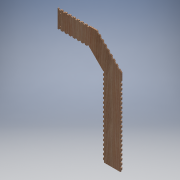
# Autodesk Inventor part: Leg
Saved by Autodesk Inventor 2019 (Build 230136000, 136)
## iProperties
Created: 2019-01-14
Part Number: Leg
Material: Wood (Birch)
Document SubType Name: Modeling
Designer: nxgam
Density: 0.55 g/cm^3
Appearance: Birch - Natural Polished
Author: nxgam
Autodesk Inventor part; units mm, degrees
(part 1 of 2)
ref_plane "YZ Plane" through (0, 0, 0) normal (1, 0, 0) x (0, 1, 0)
ref_plane "XZ Plane" through (0, 0, 0) normal (0, 1, 0) x (-1, 0, 0)
ref_plane "XY Plane" through (0, 0, 0) normal (0, 0, 1) x (1, 0, 0)
sketch "Sketch1" plane through (0, 0, 0) normal (0, 0, 1) x (1, 0, 0)
  line L0 (223.52, 0) -> (314.96, 0)
  line L1 (314.96, 0) -> (314.96, 396.2274)
  line L2 (314.96, 396.2274) -> (223.52, 396.2274)
  line L3 (223.52, 396.2274) -> (223.52, 0)
  line L4 (223.52, 396.2274) -> (154.9528, 464.7946)
  line L5 (154.9528, 464.7946) -> (219.6107, 529.4524)
  line L6 (219.6107, 529.4524) -> (314.96, 434.1031)
  line L7 (314.96, 434.1031) -> (314.96, 396.2274)
  line L8 (154.9528, 464.7946) -> (0, 464.7946)
  line L9 (0, 464.7946) -> (0, 556.2346)
  line L10 (0, 556.2346) -> (192.8285, 556.2346)
  line L11 (192.8285, 556.2346) -> (219.6107, 529.4524)
  circle A0 centre (0, 510.5146) radius 19.05
  line L12 (0, 0) -> (0, 464.7946) construction
  line L13 (0, 0) -> (223.52, 0) construction
  dimension "d0" = 91.44
  dimension "d2" = 91.44
  dimension "d3" = 135
  dimension "d4" = 91.44
  dimension "d5" = 38.1
  dimension "d6" = 556.2346
  dimension "d7" = 223.52
  dimension "d24" = 172.72
  constraints: 28 end point, 7 perpendicular, 4 collinear, 2 horizontal, 2 parallel, 2 point on line, 1 centre point, 1 midpoint
  measures "d0" distance of L2.end L1.end
  measures "d2" distance between parallel lines of L6 L4
  measures "d3" angle of L4 L3
  measures "d4" distance between parallel lines of L10 L8
  measures "d5" diameter of A0
  measures "d6" distance between parallel lines of L10 L13
  measures "d7" distance between parallel lines of L12 L3
  measures "d24" distance of L6.end L10.end
extrude "Extrusion1" add sketch "Sketch1" along normal blind 5.08 contours L3 L2 L1 L0 | L4 L5 L6 L7 L2 | L8 L9 A0 L10 L11 L5 | L9 A0 picked at (5.3722, 505.7092)
sketch "Sketch3" plane through (0, 0, 5.08) normal (0, 0, 1) x (1, 0, 0)
  line L0 (0, 464.7946) -> (154.9528, 464.7946) projected
  line L1 (0, 464.7946) -> (10.16, 464.7946)
  line L2 (10.16, 464.7946) -> (10.16, 469.8746)
  line L3 (10.16, 469.8746) -> (0, 469.8746)
  line L4 (0, 469.8746) -> (0, 464.7946)
  line L5 (192.8285, 556.2346) -> (0, 556.2346) construction
  line L6 (0, 556.2346) -> (0, 464.7946) construction
  line L7 (0, 510.5146) -> (154.9528, 510.5146) construction
  line L8 (154.9528, 510.5146) -> (154.9528, 464.7946) construction
  line L9 (192.8285, 556.2346) -> (154.9528, 464.7946) construction
  line L10 (154.9528, 464.7946) -> (223.52, 396.2274) construction
  line L11 (314.96, 0) -> (314.96, 434.1031) construction
  line L12 (223.52, 396.2274) -> (314.96, 434.1031) construction
  line L13 (314.96, 434.1031) -> (192.8285, 556.2346) construction
  line L14 (0, 556.2346) -> (0, 464.7946) construction
  line L15 (0, 464.7946) -> (154.9528, 464.7946) construction
  line L16 (154.9528, 464.7946) -> (223.52, 396.2274) construction
  line L17 (223.52, 396.2274) -> (223.52, 0) construction
  line L18 (223.52, 0) -> (314.96, 0) construction
  line L19 (314.96, 0) -> (314.96, 434.1031) construction
  line L20 (314.96, 434.1031) -> (192.8285, 556.2346) construction
  line L21 (192.8285, 556.2346) -> (0, 556.2346) construction
  line L22 (30.48, 464.7946) -> (30.48, 469.8746)
  line L23 (20.32, 464.7946) -> (30.48, 464.7946)
  line L24 (20.32, 469.8746) -> (20.32, 464.7946)
  line L25 (30.48, 469.8746) -> (20.32, 469.8746)
  line L26 (50.8, 464.7946) -> (50.8, 469.8746)
  line L27 (40.64, 464.7946) -> (50.8, 464.7946)
  line L28 (40.64, 469.8746) -> (40.64, 464.7946)
  line L29 (50.8, 469.8746) -> (40.64, 469.8746)
  line L30 (71.12, 464.7946) -> (71.12, 469.8746)
  line L31 (60.96, 464.7946) -> (71.12, 464.7946)
  line L32 (60.96, 469.8746) -> (60.96, 464.7946)
  line L33 (71.12, 469.8746) -> (60.96, 469.8746)
  line L34 (91.44, 464.7946) -> (91.44, 469.8746)
  line L35 (81.28, 464.7946) -> (91.44, 464.7946)
  line L36 (81.28, 469.8746) -> (81.28, 464.7946)
  line L37 (91.44, 469.8746) -> (81.28, 469.8746)
  line L38 (111.76, 464.7946) -> (111.76, 469.8746)
  line L39 (101.6, 464.7946) -> (111.76, 464.7946)
  line L40 (101.6, 469.8746) -> (101.6, 464.7946)
  line L41 (111.76, 469.8746) -> (101.6, 469.8746)
  line L42 (132.08, 464.7946) -> (132.08, 469.8746)
  line L43 (121.92, 464.7946) -> (132.08, 464.7946)
  line L44 (121.92, 469.8746) -> (121.92, 464.7946)
  line L45 (132.08, 469.8746) -> (121.92, 469.8746)
  line L46 (152.4, 464.7946) -> (152.4, 469.8746)
  line L47 (142.24, 464.7946) -> (152.4, 464.7946)
  line L48 (142.24, 469.8746) -> (142.24, 464.7946)
  line L49 (152.4, 469.8746) -> (142.24, 469.8746)
  line L50 (172.72, 464.7946) -> (172.72, 469.8746)
  line L51 (162.56, 464.7946) -> (172.72, 464.7946)
  line L52 (162.56, 469.8746) -> (162.56, 464.7946)
  line L53 (172.72, 469.8746) -> (162.56, 469.8746)
  line L54 (193.04, 464.7946) -> (193.04, 469.8746)
  line L55 (182.88, 464.7946) -> (193.04, 464.7946)
  line L56 (182.88, 469.8746) -> (182.88, 464.7946)
  line L57 (193.04, 469.8746) -> (182.88, 469.8746)
  line L58 (213.36, 464.7946) -> (213.36, 469.8746)
  line L59 (203.2, 464.7946) -> (213.36, 464.7946)
  line L60 (203.2, 469.8746) -> (203.2, 464.7946)
  line L61 (213.36, 469.8746) -> (203.2, 469.8746)
  line L62 (233.68, 464.7946) -> (233.68, 469.8746)
  line L63 (223.52, 464.7946) -> (233.68, 464.7946)
  line L64 (223.52, 469.8746) -> (223.52, 464.7946)
  line L65 (233.68, 469.8746) -> (223.52, 469.8746)
  line L66 (0, 556.2346) -> (10.16, 556.2346)
  line L67 (10.16, 556.2346) -> (10.16, 551.1546)
  line L68 (10.16, 551.1546) -> (0, 551.1546)
  line L69 (0, 551.1546) -> (0, 556.2346)
  line L70 (30.48, 556.2346) -> (30.48, 551.1546)
  line L71 (20.32, 556.2346) -> (30.48, 556.2346)
  line L72 (20.32, 551.1546) -> (20.32, 556.2346)
  line L73 (30.48, 551.1546) -> (20.32, 551.1546)
  line L74 (50.8, 556.2346) -> (50.8, 551.1546)
  line L75 (40.64, 556.2346) -> (50.8, 556.2346)
  line L76 (40.64, 551.1546) -> (40.64, 556.2346)
  line L77 (50.8, 551.1546) -> (40.64, 551.1546)
  line L78 (71.12, 556.2346) -> (71.12, 551.1546)
  line L79 (60.96, 556.2346) -> (71.12, 556.2346)
  line L80 (60.96, 551.1546) -> (60.96, 556.2346)
  line L81 (71.12, 551.1546) -> (60.96, 551.1546)
  line L82 (91.44, 556.2346) -> (91.44, 551.1546)
  line L83 (81.28, 556.2346) -> (91.44, 556.2346)
  line L84 (81.28, 551.1546) -> (81.28, 556.2346)
  line L85 (91.44, 551.1546) -> (81.28, 551.1546)
  line L86 (111.76, 556.2346) -> (111.76, 551.1546)
  line L87 (101.6, 556.2346) -> (111.76, 556.2346)
  line L88 (101.6, 551.1546) -> (101.6, 556.2346)
  line L89 (111.76, 551.1546) -> (101.6, 551.1546)
  line L90 (132.08, 556.2346) -> (132.08, 551.1546)
  line L91 (121.92, 556.2346) -> (132.08, 556.2346)
  line L92 (121.92, 551.1546) -> (121.92, 556.2346)
  line L93 (132.08, 551.1546) -> (121.92, 551.1546)
  line L94 (152.4, 556.2346) -> (152.4, 551.1546)
  line L95 (142.24, 556.2346) -> (152.4, 556.2346)
  line L96 (142.24, 551.1546) -> (142.24, 556.2346)
  line L97 (152.4, 551.1546) -> (142.24, 551.1546)
  line L98 (172.72, 556.2346) -> (172.72, 551.1546)
  line L99 (162.56, 556.2346) -> (172.72, 556.2346)
  line L100 (162.56, 551.1546) -> (162.56, 556.2346)
  line L101 (172.72, 551.1546) -> (162.56, 551.1546)
  line L102 (193.04, 556.2346) -> (193.04, 551.1546)
  line L103 (182.88, 556.2346) -> (193.04, 556.2346)
  line L104 (182.88, 551.1546) -> (182.88, 556.2346)
  line L105 (193.04, 551.1546) -> (182.88, 551.1546)
  line L106 (213.36, 556.2346) -> (213.36, 551.1546)
  line L107 (203.2, 556.2346) -> (213.36, 556.2346)
  line L108 (203.2, 551.1546) -> (203.2, 556.2346)
  line L109 (213.36, 551.1546) -> (203.2, 551.1546)
  line L110 (233.68, 556.2346) -> (233.68, 551.1546)
  line L111 (223.52, 556.2346) -> (233.68, 556.2346)
  line L112 (223.52, 551.1546) -> (223.52, 556.2346)
  line L113 (233.68, 551.1546) -> (223.52, 551.1546)
  line L114 (223.52, 0) -> (314.96, 0) construction
  line L115 (269.24, 0) -> (269.24, 396.2274) construction
  line L116 (269.24, 396.2274) -> (223.52, 396.2274) construction
  line L117 (223.52, 396.2274) -> (228.6, 396.2274)
  line L118 (228.6, 396.2274) -> (228.6, 386.0674)
  line L119 (228.6, 386.0674) -> (223.52, 386.0674)
  line L120 (223.52, 386.0674) -> (223.52, 396.2274)
  line L121 (223.52, 375.9074) -> (228.6, 375.9074)
  line L122 (228.6, 375.9074) -> (228.6, 365.7474)
  line L123 (228.6, 365.7474) -> (223.52, 365.7474)
  line L124 (223.52, 365.7474) -> (223.52, 375.9074)
  line L125 (223.52, 355.5874) -> (228.6, 355.5874)
  line L126 (228.6, 355.5874) -> (228.6, 345.4274)
  line L127 (228.6, 345.4274) -> (223.52, 345.4274)
  line L128 (223.52, 345.4274) -> (223.52, 355.5874)
  line L129 (223.52, 335.2674) -> (228.6, 335.2674)
  line L130 (228.6, 335.2674) -> (228.6, 325.1074)
  line L131 (228.6, 325.1074) -> (223.52, 325.1074)
  line L132 (223.52, 325.1074) -> (223.52, 335.2674)
  line L133 (223.52, 314.9474) -> (228.6, 314.9474)
  line L134 (228.6, 314.9474) -> (228.6, 304.7874)
  line L135 (228.6, 304.7874) -> (223.52, 304.7874)
  line L136 (223.52, 304.7874) -> (223.52, 314.9474)
  line L137 (223.52, 294.6274) -> (228.6, 294.6274)
  line L138 (228.6, 294.6274) -> (228.6, 284.4674)
  line L139 (228.6, 284.4674) -> (223.52, 284.4674)
  line L140 (223.52, 284.4674) -> (223.52, 294.6274)
  line L141 (223.52, 274.3074) -> (228.6, 274.3074)
  line L142 (228.6, 274.3074) -> (228.6, 264.1474)
  line L143 (228.6, 264.1474) -> (223.52, 264.1474)
  line L144 (223.52, 264.1474) -> (223.52, 274.3074)
  line L145 (223.52, 253.9874) -> (228.6, 253.9874)
  line L146 (228.6, 253.9874) -> (228.6, 243.8274)
  line L147 (228.6, 243.8274) -> (223.52, 243.8274)
  line L148 (223.52, 243.8274) -> (223.52, 253.9874)
  line L149 (223.52, 233.6674) -> (228.6, 233.6674)
  line L150 (228.6, 233.6674) -> (228.6, 223.5074)
  line L151 (228.6, 223.5074) -> (223.52, 223.5074)
  line L152 (223.52, 223.5074) -> (223.52, 233.6674)
  line L153 (223.52, 213.3474) -> (228.6, 213.3474)
  line L154 (228.6, 213.3474) -> (228.6, 203.1874)
  line L155 (228.6, 203.1874) -> (223.52, 203.1874)
  line L156 (223.52, 203.1874) -> (223.52, 213.3474)
  line L157 (223.52, 193.0274) -> (228.6, 193.0274)
  line L158 (228.6, 193.0274) -> (228.6, 182.8674)
  line L159 (228.6, 182.8674) -> (223.52, 182.8674)
  line L160 (223.52, 182.8674) -> (223.52, 193.0274)
  line L161 (223.52, 172.7074) -> (228.6, 172.7074)
  line L162 (228.6, 172.7074) -> (228.6, 162.5474)
  line L163 (228.6, 162.5474) -> (223.52, 162.5474)
  line L164 (223.52, 162.5474) -> (223.52, 172.7074)
  line L165 (223.52, 152.3874) -> (228.6, 152.3874)
  line L166 (228.6, 152.3874) -> (228.6, 142.2274)
  line L167 (228.6, 142.2274) -> (223.52, 142.2274)
  line L168 (223.52, 142.2274) -> (223.52, 152.3874)
  line L169 (223.52, 132.0674) -> (228.6, 132.0674)
  line L170 (228.6, 132.0674) -> (228.6, 121.9074)
  line L171 (228.6, 121.9074) -> (223.52, 121.9074)
  line L172 (223.52, 121.9074) -> (223.52, 132.0674)
  line L173 (223.52, 111.7474) -> (228.6, 111.7474)
  line L174 (228.6, 111.7474) -> (228.6, 101.5874)
  line L175 (228.6, 101.5874) -> (223.52, 101.5874)
  line L176 (223.52, 101.5874) -> (223.52, 111.7474)
  line L177 (223.52, 91.4274) -> (228.6, 91.4274)
  line L178 (228.6, 91.4274) -> (228.6, 81.2674)
  line L179 (228.6, 81.2674) -> (223.52, 81.2674)
  line L180 (223.52, 81.2674) -> (223.52, 91.4274)
  line L181 (314.96, 396.2274) -> (309.88, 396.2274)
  line L182 (309.88, 396.2274) -> (309.88, 386.0674)
  line L183 (309.88, 386.0674) -> (314.96, 386.0674)
  line L184 (314.96, 386.0674) -> (314.96, 396.2274)
  line L185 (314.96, 375.9074) -> (309.88, 375.9074)
  line L186 (309.88, 375.9074) -> (309.88, 365.7474)
  line L187 (309.88, 365.7474) -> (314.96, 365.7474)
  line L188 (314.96, 365.7474) -> (314.96, 375.9074)
  line L189 (314.96, 355.5874) -> (309.88, 355.5874)
  line L190 (309.88, 355.5874) -> (309.88, 345.4274)
  line L191 (309.88, 345.4274) -> (314.96, 345.4274)
  line L192 (314.96, 345.4274) -> (314.96, 355.5874)
  line L193 (314.96, 335.2674) -> (309.88, 335.2674)
  line L194 (309.88, 335.2674) -> (309.88, 325.1074)
  line L195 (309.88, 325.1074) -> (314.96, 325.1074)
  line L196 (314.96, 325.1074) -> (314.96, 335.2674)
  line L197 (314.96, 314.9474) -> (309.88, 314.9474)
  line L198 (309.88, 314.9474) -> (309.88, 304.7874)
  line L199 (309.88, 304.7874) -> (314.96, 304.7874)
  line L200 (314.96, 304.7874) -> (314.96, 314.9474)
  line L201 (314.96, 294.6274) -> (309.88, 294.6274)
  line L202 (309.88, 294.6274) -> (309.88, 284.4674)
  line L203 (309.88, 284.4674) -> (314.96, 284.4674)
  line L204 (314.96, 284.4674) -> (314.96, 294.6274)
  line L205 (314.96, 274.3074) -> (309.88, 274.3074)
  line L206 (309.88, 274.3074) -> (309.88, 264.1474)
  line L207 (309.88, 264.1474) -> (314.96, 264.1474)
  line L208 (314.96, 264.1474) -> (314.96, 274.3074)
  line L209 (314.96, 253.9874) -> (309.88, 253.9874)
  line L210 (309.88, 253.9874) -> (309.88, 243.8274)
  line L211 (309.88, 243.8274) -> (314.96, 243.8274)
  line L212 (314.96, 243.8274) -> (314.96, 253.9874)
  line L213 (314.96, 233.6674) -> (309.88, 233.6674)
  line L214 (309.88, 233.6674) -> (309.88, 223.5074)
  line L215 (309.88, 223.5074) -> (314.96, 223.5074)
  line L216 (314.96, 223.5074) -> (314.96, 233.6674)
  line L217 (314.96, 213.3474) -> (309.88, 213.3474)
  line L218 (309.88, 213.3474) -> (309.88, 203.1874)
  line L219 (309.88, 203.1874) -> (314.96, 203.1874)
  line L220 (314.96, 203.1874) -> (314.96, 213.3474)
  line L221 (314.96, 193.0274) -> (309.88, 193.0274)
  line L222 (309.88, 193.0274) -> (309.88, 182.8674)
  line L223 (309.88, 182.8674) -> (314.96, 182.8674)
  line L224 (314.96, 182.8674) -> (314.96, 193.0274)
  line L225 (314.96, 172.7074) -> (309.88, 172.7074)
  line L226 (309.88, 172.7074) -> (309.88, 162.5474)
  line L227 (309.88, 162.5474) -> (314.96, 162.5474)
  line L228 (314.96, 162.5474) -> (314.96, 172.7074)
  line L229 (314.96, 152.3874) -> (309.88, 152.3874)
  line L230 (309.88, 152.3874) -> (309.88, 142.2274)
  line L231 (309.88, 142.2274) -> (314.96, 142.2274)
  line L232 (314.96, 142.2274) -> (314.96, 152.3874)
  line L233 (314.96, 132.0674) -> (309.88, 132.0674)
  line L234 (309.88, 132.0674) -> (309.88, 121.9074)
  line L235 (309.88, 121.9074) -> (314.96, 121.9074)
  line L236 (314.96, 121.9074) -> (314.96, 132.0674)
  line L237 (314.96, 111.7474) -> (309.88, 111.7474)
  line L238 (309.88, 111.7474) -> (309.88, 101.5874)
  line L239 (309.88, 101.5874) -> (314.96, 101.5874)
  line L240 (314.96, 101.5874) -> (314.96, 111.7474)
  line L241 (314.96, 91.4274) -> (309.88, 91.4274)
  line L242 (309.88, 91.4274) -> (309.88, 81.2674)
  line L243 (309.88, 81.2674) -> (314.96, 81.2674)
  line L244 (314.96, 81.2674) -> (314.96, 91.4274)
  line L245 (196.4206, 552.6425) -> (203.6048, 545.4583)
  line L246 (203.6048, 545.4583) -> (200.0127, 541.8662)
  line L247 (200.0127, 541.8662) -> (192.8285, 549.0504)
  line L248 (192.8285, 549.0504) -> (196.4206, 552.6425)
  line L249 (207.1969, 534.682) -> (210.789, 538.2741)
  line L250 (214.3811, 527.4978) -> (207.1969, 534.682)
  line L251 (210.789, 538.2741) -> (217.9732, 531.0899)
  line L252 (217.9732, 531.0899) -> (214.3811, 527.4978)
  line L253 (221.5653, 520.3136) -> (225.1574, 523.9057)
  line L254 (228.7495, 513.1294) -> (221.5653, 520.3136)
  line L255 (225.1574, 523.9057) -> (232.3416, 516.7215)
  line L256 (232.3416, 516.7215) -> (228.7495, 513.1294)
  line L257 (235.9337, 505.9452) -> (239.5258, 509.5373)
  line L258 (243.118, 498.761) -> (235.9337, 505.9452)
  line L259 (239.5258, 509.5373) -> (246.7101, 502.3531)
  line L260 (246.7101, 502.3531) -> (243.118, 498.761)
  line L261 (250.3022, 491.5768) -> (253.8943, 495.1689)
  line L262 (257.4864, 484.3926) -> (250.3022, 491.5768)
  line L263 (253.8943, 495.1689) -> (261.0785, 487.9847)
  line L264 (261.0785, 487.9847) -> (257.4864, 484.3926)
  line L265 (264.6706, 477.2083) -> (268.2627, 480.8004)
  line L266 (271.8548, 470.0241) -> (264.6706, 477.2083)
  line L267 (268.2627, 480.8004) -> (275.4469, 473.6162)
  line L268 (275.4469, 473.6162) -> (271.8548, 470.0241)
  line L269 (279.039, 462.8399) -> (282.6311, 466.432)
  line L270 (286.2232, 455.6557) -> (279.039, 462.8399)
  line L271 (282.6311, 466.432) -> (289.8153, 459.2478)
  line L272 (289.8153, 459.2478) -> (286.2232, 455.6557)
  line L273 (293.4074, 448.4715) -> (296.9995, 452.0636)
  line L274 (300.5916, 441.2873) -> (293.4074, 448.4715)
  line L275 (296.9995, 452.0636) -> (304.1837, 444.8794)
  line L276 (304.1837, 444.8794) -> (300.5916, 441.2873)
  point P0 (0, 0)
  point P1 (0, 556.2346)
  point P2 (207.1969, 541.8662)
  point P3 (207.1969, 541.8662)
  point P4 (207.1969, 541.8662)
  point P5 (207.1969, 541.8662)
  point P6 (221.5653, 527.4978)
  point P7 (221.5653, 527.4978)
  point P8 (221.5653, 527.4978)
  point P9 (221.5653, 527.4978)
  point P10 (235.9337, 513.1294)
  point P11 (235.9337, 513.1294)
  point P12 (235.9337, 513.1294)
  point P13 (235.9337, 513.1294)
  point P14 (250.3022, 498.761)
  point P15 (250.3022, 498.761)
  point P16 (250.3022, 498.761)
  point P17 (250.3022, 498.761)
  point P18 (264.6706, 484.3926)
  point P19 (264.6706, 484.3926)
  point P20 (264.6706, 484.3926)
  point P21 (264.6706, 484.3926)
  point P22 (279.039, 470.0241)
  point P23 (279.039, 470.0241)
  point P24 (279.039, 470.0241)
  point P25 (279.039, 470.0241)
  point P26 (293.4074, 455.6557)
  point P27 (293.4074, 455.6557)
  point P28 (293.4074, 455.6557)
  point P29 (293.4074, 455.6557)
  dimension "d14" = 10.16
  dimension "d15" = 5.08
  dimension "d18" = 20.32
  dimension "d34" = 5.08
  dimension "d35" = 10.16
  dimension "d38" = 20.32
  dimension "d47" = 5.08
  dimension "d48" = 10.16
  dimension "d49" = 5.08
  dimension "d52" = 20.32
  constraints: 528 end point, 125 symmetric about line, 6 parallel, 6 perpendicular, 4 horizontal, 2 midpoint, 2 point on line, 2 vertical, 304 other
  measures "d14" distance of L3.end L2.end
  measures "d15" distance of L2.end L1.end
  measures "d18" distance of L0.start L23.start
  measures "d34" distance of L118.end L119.end
  measures "d35" distance of L117.end L118.end
  measures "d38" distance of L16.end L121.start
  measures "d47" distance of L245.end L246.end
  measures "d48" distance of L246.end L247.end
  measures "d49" distance from line of L20.end L248
  measures "d52" distance of L13.end point (207.197, 541.866)
extrude "Extrusion3" cut sketch "Sketch3" against normal blind 5.08
thicken "Thicken1" operation add thickness 5.08 both sides no extend neighbours yes toward (-1, 0, 0) faces at (0, 524.0613, 1.6933)
sketch "Sketch5" plane through (0, 0, 5.08) normal (0, 0, 1) x (1, 0, 0)
  line L0 (279.039, 462.8399) -> (282.6311, 466.432) projected
  line L1 (282.6311, 466.432) -> (275.4469, 473.6162) projected
  line L2 (275.4469, 473.6162) -> (271.8548, 470.0241) projected
  line L3 (271.8548, 470.0241) -> (264.6706, 477.2083) projected
  line L4 (264.6706, 477.2083) -> (268.2627, 480.8004) projected
  line L5 (268.2627, 480.8004) -> (261.0785, 487.9847) projected
  line L6 (261.0785, 487.9847) -> (257.4864, 484.3926) projected
  line L7 (257.4864, 484.3926) -> (250.3022, 491.5768) projected
  line L8 (250.3022, 491.5768) -> (253.8943, 495.1689) projected
  line L9 (253.8943, 495.1689) -> (246.7101, 502.3531) projected
  line L10 (246.7101, 502.3531) -> (243.118, 498.761) projected
  line L11 (243.118, 498.761) -> (235.9337, 505.9452) projected
  line L12 (235.9337, 505.9452) -> (239.5258, 509.5373) projected
  line L13 (239.5258, 509.5373) -> (232.3416, 516.7215) projected
  line L14 (232.3416, 516.7215) -> (228.7495, 513.1294) projected
  line L15 (228.7495, 513.1294) -> (221.5653, 520.3136) projected
  line L16 (221.5653, 520.3136) -> (225.1574, 523.9057) projected
  line L17 (225.1574, 523.9057) -> (217.9732, 531.0899) projected
  line L18 (217.9732, 531.0899) -> (214.3811, 527.4978) projected
  line L19 (214.3811, 527.4978) -> (207.1969, 534.682) projected
  line L20 (207.1969, 534.682) -> (210.789, 538.2741) projected
  line L21 (210.789, 538.2741) -> (203.6048, 545.4583) projected
  line L22 (203.6048, 545.4583) -> (200.0127, 541.8662) projected
  line L23 (200.0127, 541.8662) -> (192.8285, 549.0504) projected
  line L24 (192.8285, 549.0504) -> (196.4206, 552.6425) projected
  line L25 (196.4206, 552.6425) -> (193.04, 556.0231) projected
  line L26 (193.04, 556.0231) -> (193.04, 551.1546) projected
  line L27 (193.04, 551.1546) -> (182.88, 551.1546) projected
  line L28 (182.88, 551.1546) -> (182.88, 556.2346) projected
  line L29 (182.88, 556.2346) -> (172.72, 556.2346) projected
  line L30 (172.72, 556.2346) -> (172.72, 551.1546) projected
  line L31 (172.72, 551.1546) -> (162.56, 551.1546) projected
  line L32 (162.56, 551.1546) -> (162.56, 556.2346) projected
  line L33 (162.56, 556.2346) -> (152.4, 556.2346) projected
  line L34 (152.4, 556.2346) -> (152.4, 551.1546) projected
  line L35 (152.4, 551.1546) -> (142.24, 551.1546) projected
  line L36 (142.24, 551.1546) -> (142.24, 556.2346) projected
  line L37 (142.24, 556.2346) -> (132.08, 556.2346) projected
  line L38 (132.08, 556.2346) -> (132.08, 551.1546) projected
  line L39 (132.08, 551.1546) -> (121.92, 551.1546) projected
  line L40 (121.92, 551.1546) -> (121.92, 556.2346) projected
  line L41 (121.92, 556.2346) -> (111.76, 556.2346) projected
  line L42 (111.76, 556.2346) -> (111.76, 551.1546) projected
  line L43 (111.76, 551.1546) -> (101.6, 551.1546) projected
  line L44 (101.6, 551.1546) -> (101.6, 556.2346) projected
  line L45 (101.6, 556.2346) -> (91.44, 556.2346) projected
  line L46 (91.44, 556.2346) -> (91.44, 551.1546) projected
  line L47 (91.44, 551.1546) -> (81.28, 551.1546) projected
  line L48 (81.28, 551.1546) -> (81.28, 556.2346) projected
  line L49 (81.28, 556.2346) -> (71.12, 556.2346) projected
  line L50 (71.12, 556.2346) -> (71.12, 551.1546) projected
  line L51 (71.12, 551.1546) -> (60.96, 551.1546) projected
  line L52 (60.96, 551.1546) -> (60.96, 556.2346) projected
  line L53 (60.96, 556.2346) -> (50.8, 556.2346) projected
  line L54 (50.8, 556.2346) -> (50.8, 551.1546) projected
  line L55 (50.8, 551.1546) -> (40.64, 551.1546) projected
  line L56 (40.64, 551.1546) -> (40.64, 556.2346) projected
  line L57 (40.64, 556.2346) -> (30.48, 556.2346) projected
  line L58 (30.48, 556.2346) -> (30.48, 551.1546) projected
  line L59 (30.48, 551.1546) -> (20.32, 551.1546) projected
  line L60 (20.32, 551.1546) -> (20.32, 556.2346) projected
  line L61 (20.32, 556.2346) -> (10.16, 556.2346) projected
  line L62 (10.16, 556.2346) -> (10.16, 551.1546) projected
  line L63 (10.16, 551.1546) -> (-5.08, 551.1546) projected
  line L64 (-5.08, 551.1546) -> (-5.08, 469.8746) projected
  line L65 (-5.08, 469.8746) -> (10.16, 469.8746) projected
  line L66 (10.16, 469.8746) -> (10.16, 464.7946) projected
  line L67 (10.16, 464.7946) -> (20.32, 464.7946) projected
  line L68 (20.32, 464.7946) -> (20.32, 469.8746) projected
  line L69 (20.32, 469.8746) -> (30.48, 469.8746) projected
  line L70 (30.48, 469.8746) -> (30.48, 464.7946) projected
  line L71 (30.48, 464.7946) -> (40.64, 464.7946) projected
  line L72 (40.64, 464.7946) -> (40.64, 469.8746) projected
  line L73 (40.64, 469.8746) -> (50.8, 469.8746) projected
  line L74 (50.8, 469.8746) -> (50.8, 464.7946) projected
  line L75 (50.8, 464.7946) -> (60.96, 464.7946) projected
  line L76 (60.96, 464.7946) -> (60.96, 469.8746) projected
  line L77 (60.96, 469.8746) -> (71.12, 469.8746) projected
  line L78 (71.12, 469.8746) -> (71.12, 464.7946) projected
  line L79 (71.12, 464.7946) -> (81.28, 464.7946) projected
  line L80 (81.28, 464.7946) -> (81.28, 469.8746) projected
  line L81 (81.28, 469.8746) -> (91.44, 469.8746) projected
  line L82 (91.44, 469.8746) -> (91.44, 464.7946) projected
  line L83 (91.44, 464.7946) -> (101.6, 464.7946) projected
  line L84 (101.6, 464.7946) -> (101.6, 469.8746) projected
  line L85 (101.6, 469.8746) -> (111.76, 469.8746) projected
  line L86 (111.76, 469.8746) -> (111.76, 464.7946) projected
  line L87 (111.76, 464.7946) -> (121.92, 464.7946) projected
  line L88 (121.92, 464.7946) -> (121.92, 469.8746) projected
  line L89 (121.92, 469.8746) -> (132.08, 469.8746) projected
  line L90 (132.08, 469.8746) -> (132.08, 464.7946) projected
  line L91 (132.08, 464.7946) -> (142.24, 464.7946) projected
  line L92 (142.24, 464.7946) -> (142.24, 469.8746) projected
  line L93 (142.24, 469.8746) -> (152.4, 469.8746) projected
  line L94 (152.4, 469.8746) -> (152.4, 464.7946) projected
  line L95 (152.4, 464.7946) -> (154.9528, 464.7946) projected
  line L96 (162.56, 464.7946) -> (162.56, 469.8746) projected
  line L97 (162.56, 469.8746) -> (172.72, 469.8746) projected
  line L98 (172.72, 469.8746) -> (172.72, 464.7946) projected
  line L99 (182.88, 464.7946) -> (182.88, 469.8746) projected
  line L100 (182.88, 469.8746) -> (193.04, 469.8746) projected
  line L101 (193.04, 469.8746) -> (193.04, 464.7946) projected
  line L102 (203.2, 464.7946) -> (203.2, 469.8746) projected
  line L103 (203.2, 469.8746) -> (213.36, 469.8746) projected
  line L104 (213.36, 469.8746) -> (213.36, 464.7946) projected
  line L105 (223.52, 464.7946) -> (223.52, 469.8746) projected
  line L106 (223.52, 469.8746) -> (233.68, 469.8746) projected
  line L107 (233.68, 469.8746) -> (233.68, 464.7946) projected
  line L108 (154.9528, 464.7946) -> (223.52, 396.2274) projected
  line L109 (223.52, 396.2274) -> (228.6, 396.2274) projected
  line L110 (228.6, 396.2274) -> (228.6, 386.0674) projected
  line L111 (228.6, 386.0674) -> (223.52, 386.0674) projected
  line L112 (223.52, 386.0674) -> (223.52, 375.9074) projected
  line L113 (223.52, 375.9074) -> (228.6, 375.9074) projected
  line L114 (228.6, 375.9074) -> (228.6, 365.7474) projected
  line L115 (228.6, 365.7474) -> (223.52, 365.7474) projected
  line L116 (223.52, 365.7474) -> (223.52, 355.5874) projected
  line L117 (223.52, 355.5874) -> (228.6, 355.5874) projected
  line L118 (228.6, 355.5874) -> (228.6, 345.4274) projected
  line L119 (228.6, 345.4274) -> (223.52, 345.4274) projected
  line L120 (223.52, 345.4274) -> (223.52, 335.2674) projected
  line L121 (223.52, 335.2674) -> (228.6, 335.2674) projected
  line L122 (228.6, 335.2674) -> (228.6, 325.1074) projected
  line L123 (228.6, 325.1074) -> (223.52, 325.1074) projected
  line L124 (223.52, 325.1074) -> (223.52, 314.9474) projected
  line L125 (223.52, 314.9474) -> (228.6, 314.9474) projected
  line L126 (228.6, 314.9474) -> (228.6, 304.7874) projected
  line L127 (228.6, 304.7874) -> (223.52, 304.7874) projected
  line L128 (223.52, 304.7874) -> (223.52, 294.6274) projected
  line L129 (223.52, 294.6274) -> (228.6, 294.6274) projected
  line L130 (228.6, 294.6274) -> (228.6, 284.4674) projected
  line L131 (228.6, 284.4674) -> (223.52, 284.4674) projected
  line L132 (223.52, 284.4674) -> (223.52, 274.3074) projected
  line L133 (223.52, 274.3074) -> (228.6, 274.3074) projected
  line L134 (228.6, 274.3074) -> (228.6, 264.1474) projected
  line L135 (228.6, 264.1474) -> (223.52, 264.1474) projected
  line L136 (223.52, 264.1474) -> (223.52, 253.9874) projected
  line L137 (223.52, 253.9874) -> (228.6, 253.9874) projected
  line L138 (228.6, 253.9874) -> (228.6, 243.8274) projected
  line L139 (228.6, 243.8274) -> (223.52, 243.8274) projected
  line L140 (223.52, 243.8274) -> (223.52, 233.6674) projected
  line L141 (223.52, 233.6674) -> (228.6, 233.6674) projected
  line L142 (228.6, 233.6674) -> (228.6, 223.5074) projected
  line L143 (228.6, 223.5074) -> (223.52, 223.5074) projected
  line L144 (223.52, 223.5074) -> (223.52, 213.3474) projected
  line L145 (223.52, 213.3474) -> (228.6, 213.3474) projected
  line L146 (228.6, 213.3474) -> (228.6, 203.1874) projected
  line L147 (228.6, 203.1874) -> (223.52, 203.1874) projected
  line L148 (223.52, 203.1874) -> (223.52, 193.0274) projected
  line L149 (223.52, 193.0274) -> (228.6, 193.0274) projected
  line L150 (228.6, 193.0274) -> (228.6, 182.8674) projected
  line L151 (228.6, 182.8674) -> (223.52, 182.8674) projected
  line L152 (223.52, 182.8674) -> (223.52, 172.7074) projected
  line L153 (223.52, 172.7074) -> (228.6, 172.7074) projected
  line L154 (228.6, 172.7074) -> (228.6, 162.5474) projected
  line L155 (228.6, 162.5474) -> (223.52, 162.5474) projected
  line L156 (223.52, 162.5474) -> (223.52, 152.3874) projected
  line L157 (223.52, 152.3874) -> (228.6, 152.3874) projected
  line L158 (228.6, 152.3874) -> (228.6, 142.2274) projected
  line L159 (228.6, 142.2274) -> (223.52, 142.2274) projected
  line L160 (223.52, 142.2274) -> (223.52, 132.0674) projected
  line L161 (223.52, 132.0674) -> (228.6, 132.0674) projected
  line L162 (228.6, 132.0674) -> (228.6, 121.9074) projected
  line L163 (228.6, 121.9074) -> (223.52, 121.9074) projected
  line L164 (223.52, 121.9074) -> (223.52, 111.7474) projected
  line L165 (223.52, 111.7474) -> (228.6, 111.7474) projected
  line L166 (228.6, 111.7474) -> (228.6, 101.5874) projected
  line L167 (228.6, 101.5874) -> (223.52, 101.5874) projected
  line L168 (223.52, 101.5874) -> (223.52, 91.4274) projected
  line L169 (223.52, 91.4274) -> (228.6, 91.4274) projected
  line L170 (228.6, 91.4274) -> (228.6, 81.2674) projected
  line L171 (228.6, 81.2674) -> (223.52, 81.2674) projected
  line L172 (223.52, 81.2674) -> (223.52, 0) projected
  line L173 (223.52, 0) -> (314.96, 0) projected
  line L174 (314.96, 0) -> (314.96, 81.2674) projected
  line L175 (314.96, 81.2674) -> (309.88, 81.2674) projected
  line L176 (309.88, 81.2674) -> (309.88, 91.4274) projected
  line L177 (309.88, 91.4274) -> (314.96, 91.4274) projected
  line L178 (314.96, 91.4274) -> (314.96, 101.5874) projected
  line L179 (314.96, 101.5874) -> (309.88, 101.5874) projected
  line L180 (309.88, 101.5874) -> (309.88, 111.7474) projected
  line L181 (309.88, 111.7474) -> (314.96, 111.7474) projected
  line L182 (314.96, 111.7474) -> (314.96, 121.9074) projected
  line L183 (314.96, 121.9074) -> (309.88, 121.9074) projected
  line L184 (309.88, 121.9074) -> (309.88, 132.0674) projected
  line L185 (309.88, 132.0674) -> (314.96, 132.0674) projected
  line L186 (314.96, 132.0674) -> (314.96, 142.2274) projected
  line L187 (314.96, 142.2274) -> (309.88, 142.2274) projected
  line L188 (309.88, 142.2274) -> (309.88, 152.3874) projected
  line L189 (309.88, 152.3874) -> (314.96, 152.3874) projected
  line L190 (314.96, 152.3874) -> (314.96, 162.5474) projected
  line L191 (314.96, 162.5474) -> (309.88, 162.5474) projected
  line L192 (309.88, 162.5474) -> (309.88, 172.7074) projected
  line L193 (309.88, 172.7074) -> (314.96, 172.7074) projected
  line L194 (314.96, 172.7074) -> (314.96, 182.8674) projected
  line L195 (314.96, 182.8674) -> (309.88, 182.8674) projected
  line L196 (309.88, 182.8674) -> (309.88, 193.0274) projected
  line L197 (309.88, 193.0274) -> (314.96, 193.0274) projected
  line L198 (314.96, 193.0274) -> (314.96, 203.1874) projected
  line L199 (314.96, 203.1874) -> (309.88, 203.1874) projected
  line L200 (309.88, 203.1874) -> (309.88, 213.3474) projected
  line L201 (309.88, 213.3474) -> (314.96, 213.3474) projected
  line L202 (314.96, 213.3474) -> (314.96, 223.5074) projected
  line L203 (314.96, 223.5074) -> (309.88, 223.5074) projected
  line L204 (309.88, 223.5074) -> (309.88, 233.6674) projected
  line L205 (309.88, 233.6674) -> (314.96, 233.6674) projected
  line L206 (314.96, 233.6674) -> (314.96, 243.8274) projected
  line L207 (314.96, 243.8274) -> (309.88, 243.8274) projected
  line L208 (309.88, 243.8274) -> (309.88, 253.9874) projected
  line L209 (309.88, 253.9874) -> (314.96, 253.9874) projected
  line L210 (314.96, 253.9874) -> (314.96, 264.1474) projected
  line L211 (314.96, 264.1474) -> (309.88, 264.1474) projected
  line L212 (309.88, 264.1474) -> (309.88, 274.3074) projected
  line L213 (309.88, 274.3074) -> (314.96, 274.3074) projected
  line L214 (314.96, 274.3074) -> (314.96, 284.4674) projected
  line L215 (314.96, 284.4674) -> (309.88, 284.4674) projected
  line L216 (309.88, 284.4674) -> (309.88, 294.6274) projected
  line L217 (309.88, 294.6274) -> (314.96, 294.6274) projected
  line L218 (314.96, 294.6274) -> (314.96, 304.7874) projected
  line L219 (314.96, 304.7874) -> (309.88, 304.7874) projected
  line L220 (309.88, 304.7874) -> (309.88, 314.9474) projected
  line L221 (309.88, 314.9474) -> (314.96, 314.9474) projected
  line L222 (314.96, 314.9474) -> (314.96, 325.1074) projected
  line L223 (314.96, 325.1074) -> (309.88, 325.1074) projected
  line L224 (309.88, 325.1074) -> (309.88, 335.2674) projected
  line L225 (309.88, 335.2674) -> (314.96, 335.2674) projected
  line L226 (314.96, 335.2674) -> (314.96, 345.4274) projected
  line L227 (314.96, 345.4274) -> (309.88, 345.4274) projected
  line L228 (309.88, 345.4274) -> (309.88, 355.5874) projected
  line L229 (309.88, 355.5874) -> (314.96, 355.5874) projected
  line L230 (314.96, 355.5874) -> (314.96, 365.7474) projected
  line L231 (314.96, 365.7474) -> (309.88, 365.7474) projected
  line L232 (309.88, 365.7474) -> (309.88, 375.9074) projected
  line L233 (309.88, 375.9074) -> (314.96, 375.9074) projected
  line L234 (314.96, 375.9074) -> (314.96, 386.0674) projected
  line L235 (314.96, 386.0674) -> (309.88, 386.0674) projected
  line L236 (309.88, 386.0674) -> (309.88, 396.2274) projected
  line L237 (309.88, 396.2274) -> (314.96, 396.2274) projected
  line L238 (314.96, 396.2274) -> (314.96, 434.1031) projected
  line L239 (314.96, 434.1031) -> (304.1837, 444.8794) projected
  line L240 (304.1837, 444.8794) -> (300.5916, 441.2873) projected
  line L241 (300.5916, 441.2873) -> (293.4074, 448.4715) projected
  line L242 (293.4074, 448.4715) -> (296.9995, 452.0636) projected
  line L243 (296.9995, 452.0636) -> (289.8153, 459.2478) projected
  line L244 (289.8153, 459.2478) -> (286.2232, 455.6557) projected
  line L245 (286.2232, 455.6557) -> (279.039, 462.8399) projected
  line L246 (228.6, 91.4274) -> (223.52, 91.4274)
  line L247 (223.52, 91.4274) -> (223.52, 81.2674)
  line L248 (223.52, 81.2674) -> (228.6, 81.2674)
  line L249 (228.6, 81.2674) -> (228.6, 91.4274)
  line L250 (228.6, 71.1074) -> (223.52, 71.1074)
  line L251 (228.6, 60.9474) -> (228.6, 71.1074)
  line L252 (223.52, 71.1074) -> (223.52, 60.9474)
  line L253 (223.52, 60.9474) -> (228.6, 60.9474)
  line L254 (228.6, 50.7874) -> (223.52, 50.7874)
  line L255 (228.6, 40.6274) -> (228.6, 50.7874)
  line L256 (223.52, 50.7874) -> (223.52, 40.6274)
  line L257 (223.52, 40.6274) -> (228.6, 40.6274)
  line L258 (228.6, 30.4674) -> (223.52, 30.4674)
  line L259 (228.6, 20.3074) -> (228.6, 30.4674)
  line L260 (223.52, 30.4674) -> (223.52, 20.3074)
  line L261 (223.52, 20.3074) -> (228.6, 20.3074)
  line L262 (228.6, 10.1474) -> (223.52, 10.1474)
  line L263 (228.6, -0.0126) -> (228.6, 10.1474)
  line L264 (223.52, 10.1474) -> (223.52, -0.0126)
  line L265 (223.52, -0.0126) -> (228.6, -0.0126)
  line L266 (228.6, -10.1726) -> (223.52, -10.1726)
  line L267 (228.6, -20.3326) -> (228.6, -10.1726)
  line L268 (223.52, -10.1726) -> (223.52, -20.3326)
  line L269 (223.52, -20.3326) -> (228.6, -20.3326)
  line L270 (223.52, 0) -> (314.96, 0) construction
  line L271 (269.24, 0) -> (269.24, 95.2938) construction
  line L272 (314.96, 101.5874) -> (314.96, 91.4274)
  line L273 (314.96, 91.4274) -> (309.88, 91.4274)
  line L274 (309.88, 91.4274) -> (309.88, 81.2674)
  line L275 (309.88, 81.2674) -> (314.96, 81.2674)
  line L276 (314.96, 81.2674) -> (314.96, 0)
  line L277 (314.96, 0) -> (223.52, 0)
  line L278 (309.88, 91.4274) -> (314.96, 91.4274)
  line L279 (314.96, 91.4274) -> (314.96, 81.2674)
  line L280 (314.96, 81.2674) -> (309.88, 81.2674)
  line L281 (309.88, 81.2674) -> (309.88, 91.4274)
  line L282 (309.88, 71.1074) -> (314.96, 71.1074)
  line L283 (309.88, 60.9474) -> (309.88, 71.1074)
  line L284 (314.96, 71.1074) -> (314.96, 60.9474)
  line L285 (314.96, 60.9474) -> (309.88, 60.9474)
  line L286 (309.88, 50.7874) -> (314.96, 50.7874)
  line L287 (309.88, 40.6274) -> (309.88, 50.7874)
  line L288 (314.96, 50.7874) -> (314.96, 40.6274)
  line L289 (314.96, 40.6274) -> (309.88, 40.6274)
  line L290 (309.88, 30.4674) -> (314.96, 30.4674)
  line L291 (309.88, 20.3074) -> (309.88, 30.4674)
  line L292 (314.96, 30.4674) -> (314.96, 20.3074)
  line L293 (314.96, 20.3074) -> (309.88, 20.3074)
  line L294 (309.88, 10.1474) -> (314.96, 10.1474)
  line L295 (309.88, -0.0126) -> (309.88, 10.1474)
  line L296 (314.96, 10.1474) -> (314.96, -0.0126)
  line L297 (314.96, -0.0126) -> (309.88, -0.0126)
  line L298 (314.96, 0) -> (223.52, 0) construction
  line L299 (233.68, 464.7946) -> (223.52, 464.7946) projected
  line L300 (193.04, 464.7946) -> (182.88, 464.7946) projected
  line L301 (172.72, 464.7946) -> (162.56, 464.7946) projected
  line L302 (213.36, 464.7946) -> (203.2, 464.7946) projected
  point P0 (0, 0)
  dimension "d62" = 20.32
  constraints: 104 end point, 22 symmetric about line, 2 parallel, 2 vertical, 1 horizontal, 1 midpoint, 1 perpendicular, 40 other
  measures "d62" distance of L246.end L250.end
extrude "Extrusion4" cut sketch "Sketch5" against normal blind 5.08 contours L245 L244 L243 L242 L241 L240 L239 L238 L237 L236 L235 L234 L233 L232 L231 L230 L229 L228 L227 L226 L225 L224 L223 L222 L221 L220 L219 L218 L217 L216 L215 L214 L213 L212 L211 L210 L209 L208 L207 L206 L205 L204 L203 L202 L201 L200 L199 L198 L197 L196 L195 L194 L193 L192 L191 L190 L189 L188 L187 L186 L185 L184 L183 L182 L181 L180 L179 L178 L177 L176 L175 L174 L282 L283 L285 L286 L287 L289 L290 L291 L293 L294 L295 L173 L263 L262 L172 L261 L259 L258 L257 L255 L254 L253 L251 L250 L171 L170 L169 L168 L167 L166 L165 L164 L163 L162 L161 L160 L159 L158 L157 L156 L155 L154 L153 L152 L151 L150 L149 L148 L147 L146 L145 L144 L143 L142 L141 L140 L139 L138 L137 L136 L135 L134 L133 L132 L131 L130 L129 L128 L127 L126 L125 L124 L123 L122 L121 L120 L119 L118 L117 L116 L115 L114 L113 L112 L111 L110 L109 L108 L95 L94 L93 L92 L91 L90 L89 L88 L87 L86 L85 L84 L83 L82 L81 L80 L79 L78 L77 L76 L75 L74 L73 L72 L71 L70 L69 L68 L67 L66 L65 L64 L63 L62 L61 L60 L59 L58 L57 L56 L55 L54 L53 L52 L51 L50 L49 L48 L47 L46 L45 L44 L43 L42 L41 L40 L39 L38 L37 L36 L35 L34 L33 L32 L31 L30 L29 L28 L27 L26 L25 L24 L23 L22 L21 L20 L19 L18 L17 L16 L15 L14 L13 L12 L11 L10 L9 L8 L7 L6 L5 L4 L3 L2 L1 L0 | L96 L97 L98 L301 | L99 L100 L101 L300 | L102 L103 L104 L302 | L105 L106 L107 L299 keep common part
sketch "Sketch6" plane through (0, 0, 5.08) normal (0, 0, 1) x (1, 0, 0)
  line L0 (-5.08, 551.1546) -> (-5.08, 469.8746) construction
  line L1 (-5.08, 510.5146) -> (75.665, 510.5146) construction
  line L2 (10.16, 551.1546) -> (-5.08, 551.1546) construction
  line L3 (7.62, 538.4546) -> (7.62, 482.5746) construction
  point P0 (0, 0)
  point P1 (7.62, 482.5746)
  dimension "d66" = 12.7
  dimension "d67" = 27.94
  dimension "d68" = 27.94
  dimension "d69" = 12.7
  constraints: 4 end point, 1 coincident, 1 horizontal, 1 midpoint, 1 vertical
  measures "d66" distance from line of L3.start L2
  measures "d67" distance from line of L1 L3.start
  measures "d68" distance from line of L1 point (7.62, 482.575)
  measures "d69" distance between parallel lines of L0 L3
hole "Hole1" at (7.62, 538.4546, 5.08) at (7.62, 482.5746, 5.08) direction (0, 0, -1) diameter 5 end through all